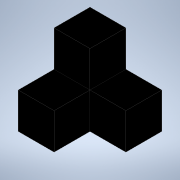
# Autodesk Inventor part: Corner
Saved by Autodesk Inventor 2020 (Build 240168000, 168)
## iProperties
Created: 2019-12-20
Part Number: Corner
Material: Generic
Document SubType Name: Modeling
Designer: Corey
Density: 1 g/cm^3
Appearance: Default
Author: Corey
Autodesk Inventor part; units mm, degrees
ref_plane "YZ Plane" through (0, 0, 0) normal (1, 0, 0) x (0, 1, 0)
ref_plane "XZ Plane" through (0, 0, 0) normal (0, 1, 0) x (-1, 0, 0)
ref_plane "XY Plane" through (0, 0, 0) normal (0, 0, 1) x (1, 0, 0)
sketch "Sketch1" plane through (0, 0, 0) normal (0, 1, 0) x (-1, 0, 0)
  line L0 (0, 0) -> (19.05, 0)
  line L1 (19.05, 0) -> (19.05, -19.05)
  line L2 (19.05, -19.05) -> (0, -19.05)
  line L3 (0, -19.05) -> (0, 0)
  line L4 (0, -19.05) -> (19.05, -19.05)
  line L5 (19.05, -19.05) -> (19.05, -38.1)
  line L6 (19.05, -38.1) -> (0, -38.1)
  line L7 (0, -38.1) -> (0, -19.05)
  line L8 (19.05, -19.05) -> (38.1, -19.05)
  line L9 (38.1, -19.05) -> (38.1, -38.1)
  line L10 (38.1, -38.1) -> (19.05, -38.1)
  line L11 (19.05, -38.1) -> (19.05, -19.05)
  dimension "d0" = 19.05
  dimension "d1" = 19.05
  dimension "d2" = 19.05
  dimension "d3" = 19.05
  dimension "d4" = 19.05
  dimension "d5" = 19.05
  constraints: 24 end point, 6 parallel, 3 horizontal, 3 perpendicular
  measures "d0" distance of L1.end L2.end
  measures "d1" distance of L0.end L1.end
  measures "d2" distance of L5.end L6.end
  measures "d3" distance of L4.end L5.end
  measures "d4" distance of L9.end L10.end
  measures "d5" distance of L8.end L9.end
extrude "Extrusion1" add sketch "Sketch1" along normal blind 19.05 contours L0 L1 L2 L3 | L8 L9 L10 L5
extrude "Extrusion2" add sketch "Sketch1" along normal blind 38.1 contours L2 L5 L6 L7
body "Solid1"
